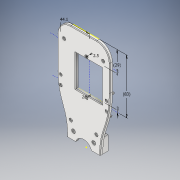
# Autodesk Inventor part: Sideplate
Saved by Autodesk Inventor 2019 (Build 230136000, 136)
## iProperties
Created: 2018-12-23
Part Number: Sideplate
Material: Generic
Document SubType Name: Modeling
Designer: Martin
Density: 1 g/cm^3
Appearance: Default
Mass: 44.7821 g
Surface Area: 242.538 cm^2
Volume: 44.7821 cm^3
Author: Martin
Autodesk Inventor part; units mm, degrees
ref_plane "YZ Plane" through (0, 0, 0) normal (1, 0, 0) x (0, 1, 0)
ref_plane "XZ Plane" through (0, 0, 0) normal (0, 1, 0) x (-1, 0, 0)
ref_plane "XY Plane" through (0, 0, 0) normal (0, 0, 1) x (1, 0, 0)
sketch "Sketch1" plane through (0, 0, 0) normal (0, 0, 1) x (1, 0, 0)
  line L0 (-21.25, 21.25) -> (21.25, 21.25)
  line L1 (21.25, 21.25) -> (21.25, -21.25)
  line L2 (21.25, -21.25) -> (-21.25, -21.25)
  line L3 (-21.25, -21.25) -> (-21.25, 21.25)
  line L4 (-21.25, 21.25) -> (21.25, -21.25) construction
  line L5 (21.25, 21.25) -> (-21.25, -21.25) construction
  circle A0 centre (0, 0) radius 11 construction
  circle A1 centre (0, 0) radius 12.5
  line L6 (-25.25, 3.5236) -> (25.25, 3.5236)
  line L7 (25.25, 3.5236) -> (25.25, 25.25)
  line L8 (25.25, 25.25) -> (-25.25, 25.25)
  line L9 (-25.25, 25.25) -> (-25.25, 3.5236)
  circle A2 centre (-15.5, 15.5) radius 1.5
  circle A3 centre (15.5, 15.5) radius 1.5
  point P0 (21.25, 3.5236)
  point P1 (-21.25, 3.5236)
  dimension "d0" = 42.5
  dimension "d1" = 42.5
  dimension "d2" = 22
  dimension "d3" = 25
  dimension "d4" = 4
  dimension "d5" = 4
  dimension "d6" = 4
  dimension "d7" = 3
  dimension "d8" = 3
  dimension "d9" = 15.5
  dimension "d10" = 15.5
  dimension "d11" = 15.5
  dimension "d12" = 15.5
  constraints: 20 end point, 4 centre point, 4 parallel, 4 point on line, 2 coincident, 2 horizontal, 2 midpoint, 2 perpendicular
  measures "d0" distance of L1.end L2.end
  measures "d1" distance of L0.end L1.end
  measures "d2" diameter of A0
  measures "d3" diameter of A1
  measures "d4" distance between parallel lines of L0 L8
  measures "d5" distance between parallel lines of L9 L3
  measures "d6" distance between parallel lines of L7 L1
  measures "d7" diameter of A3
  measures "d8" diameter of A2
  measures "d9" horizontal distance of A3.centre point (0, 0)
  measures "d10" horizontal distance of A3.centre point (0, 0)
  measures "d11" horizontal distance of A2.centre A0.centre
  measures "d12" horizontal distance of point (0, 0) A2.centre
extrude "Extrusion1" add sketch "Sketch1" along normal blind 4 contours L3 L6 L9 L8 L7 L1 L0 | L0 L1 L6 A1 L3 | A1 L6 picked at (3.04, 5.1985)
extrude "Extrusion3" add sketch "Sketch1" against normal blind 8 contours L3 L6 L9 L8 L7 L1 L0
sketch "Sketch2" plane through (0, 0, 4) normal (0, 0, 1) x (1, 0, 0)
  circle A0 centre (0, 0) radius 40 construction
  line L0 (-25.25, 3.5236) -> (25.25, 3.5236) construction
  line L1 (-25.25, 3.5236) -> (25.25, 3.5236) projected
  line L2 (-25.25, 3.5236) -> (25.25, 3.5236)
  line L3 (39.8445, 92.8978) -> (39.8445, 152.8119)
  line L4 (39.8445, 152.8119) -> (-39.8445, 152.8119)
  line L5 (-39.8445, 152.8119) -> (-39.8445, 82.8978)
  circle A1 centre (-15.5, 15.5) radius 1.5 projected
  circle A2 centre (-15.5, 15.5) radius 1.5
  circle A3 centre (15.5, 15.5) radius 1.5 projected
  circle A4 centre (15.5, 15.5) radius 1.5
  line L6 (25.25, 43.5236) -> (25.25, 3.5236) projected
  line L7 (25.25, 43.5236) -> (25.25, -31.0232) construction
  line L8 (-25.25, 25.25) -> (-25.25, -31.0232) construction
  line L9 (25.25, 3.5236) -> (25.25, 43.5236) projected
  line L10 (25.25, 3.5236) -> (25.25, 43.5236) construction
  line L11 (25.25, 43.5236) -> (39.8445, 43.5236) construction
  line L12 (39.8445, 43.5236) -> (39.8445, 92.8978) construction
  spline S0 degree 3 poles (25.25, 3.5236) (25.25, 43.5236) (39.8445, 43.5236) (39.8445, 92.8978) knots 1 1 1 1 2 2 2 2
  line L13 (-25.25, 3.5236) -> (-25.25, 43.5236) construction
  line L14 (-25.25, 43.5236) -> (-39.8445, 43.5236) construction
  line L15 (-39.8445, 43.5236) -> (-39.8445, 82.8978) construction
  spline S1 degree 3 poles (-25.25, 3.5236) (-25.25, 43.5236) (-39.8445, 43.5236) (-39.8445, 82.8978) knots 1 1 1 1 2 2 2 2
  line L16 (34.8445, 168.0706) -> (34.8445, -11.808) construction
  line L17 (-34.8445, 167.0543) -> (-34.8445, -11.808) construction
  line L18 (51.4064, 130.8119) -> (-51.1328, 130.8119) construction
  line L19 (29.8445, 167.0543) -> (29.8445, 90.5025) construction
  line L20 (-29.8445, 165.7121) -> (-29.8445, 89.1603) construction
  circle A5 centre (29.8445, 130.8119) radius 1.25
  circle A6 centre (-29.8445, 130.8119) radius 1.25
  point P0 (-11.9931, 3.5236)
  point P1 (-39.8445, 3.5236)
  point P2 (39.8445, 3.5236)
  dimension "d19" = 80
  dimension "d20" = 150
  dimension "d21" = 39.8445
  dimension "d33" = 40
  dimension "d34" = 40
  dimension "d35" = 40
  dimension "d36" = 39.8445
  dimension "d37" = 5
  dimension "d38" = 5
  dimension "d68" = 22
  dimension "d69" = 10
  dimension "d70" = 10
  dimension "d71" = 2.5
  dimension "d72" = 2.5
  constraints: 24 end point, 7 point on line, 5 centre point, 4 coincident, 4 collinear, 4 vertical, 3 parallel, 2 horizontal, 2 perpendicular, 2 point on circle, 8 other
  measures "d19" diameter of A0
  measures "d20" distance of L0.end L3.end
  measures "d21" distance from line of L3 A0.centre
  measures "d33" distance from line of L0 L14.end
  measures "d34" distance from line of L0 L11.end
  measures "d35" distance from line of L0 L6.start
  measures "d36" distance from line of L5 point (0, 0)
  measures "d37" distance between parallel lines of L3 L16
  measures "d38" distance between parallel lines of L5 L17
  measures "d68" distance between parallel lines of L18 L4
  measures "d69" distance between parallel lines of L19 L3
  measures "d70" distance between parallel lines of L5 L20
  measures "d71" diameter of A5
  measures "d72" diameter of A6
extrude "Extrusion4" add sketch "Sketch2" against normal blind 4 contours S1 L5 L4 L3 S0 L1 | A5 | A6
fillet "Fillet1" radius 20 2 edges at (-39.8445, 152.8119, 2) (39.8445, 152.8119, 2)
sketch "Sketch3" plane through (0, 0, 0) normal (0, 0, -1) x (-1, 0, 0)
  line L0 (-40.0079, 28.25) -> (78.3012, 28.25) construction
  line L1 (25.25, 25.25) -> (-25.25, 25.25) projected
  line L2 (-19.5, 51.7245) -> (-19.5, -25.7194) construction
  line L3 (19.5, 50.7243) -> (19.5, -26.4338) construction
  circle A0 centre (-19.5, 28.25) radius 1.25
  circle A1 centre (19.5, 28.25) radius 1.25
  point P0 (0, 0)
  dimension "d26" = 3
  dimension "d27" = 19.5
  dimension "d28" = 19.5
  dimension "d29" = 2.5
  dimension "d30" = 2.5
  constraints: 6 end point, 4 point on line, 2 centre point, 2 vertical, 1 horizontal
  measures "d26" distance between parallel lines of L0 L1
  measures "d27" distance from line of point (0, 0) L2
  measures "d28" distance from line of L3 point (0, 0)
  measures "d29" diameter of A0
  measures "d30" diameter of A1
extrude "Extrusion5" cut sketch "Sketch3" against normal blind 10
sketch "Sketch4" plane through (0, 0, 0) normal (0, 0, -1) x (-1, 0, 0)
  line L0 (-34.8445, 174.3908) -> (-34.8445, -4.6748) construction
  line L1 (34.8445, 172.891) -> (34.8445, -6.1746) construction
  line L2 (39.8445, 174.885) -> (39.8445, -4.1806) construction
  line L3 (39.8445, 82.8978) -> (39.8445, 132.8119) projected
  line L4 (-39.8445, 132.8119) -> (-39.8445, 92.8978) projected
  line L5 (-58.077, 152.8119) -> (62.4518, 152.8119) construction
  line L6 (19.8445, 152.8119) -> (-19.8445, 152.8119) projected
  line L7 (-60.7578, 80.8119) -> (59.771, 80.8119) construction
  line L8 (-61.2028, 66.8119) -> (59.326, 66.8119) construction
  circle A0 centre (-34.8445, 80.8119) radius 1
  circle A1 centre (-34.8445, 66.8119) radius 1
  circle A2 centre (34.8445, 80.8119) radius 1
  circle A3 centre (34.8445, 66.8119) radius 1
  line L9 (-29.8445, 176.1827) -> (-29.8445, -2.8829) construction
  line L10 (29.8445, 178.0117) -> (29.8445, -1.0539) construction
  line L11 (-58.5074, 88.8119) -> (62.0214, 88.8119) construction
  line L12 (-58.4589, 58.8119) -> (62.0699, 58.8119) construction
  line L13 (-39.8445, 88.8119) -> (-29.8445, 88.8119) construction
  line L14 (-29.8445, 88.8119) -> (-29.8445, 58.8119) construction
  line L15 (-29.8445, 58.8119) -> (-36.5289, 58.8119) construction
  line L16 (-36.5289, 58.7119) -> (-29.7445, 58.7119)
  line L17 (-29.7445, 58.7119) -> (-29.7445, 88.9119)
  line L18 (-29.7445, 88.9119) -> (-39.7987, 88.9119)
  line L19 (-39.8276, 90.9119) -> (-27.7445, 90.9119)
  line L20 (-27.7445, 56.7119) -> (-36.0331, 56.7119)
  line L21 (-36.5289, 58.7119) -> (-36.0331, 56.7119)
  line L22 (-39.8445, 176.1815) -> (-39.8445, 90.9119) construction
  line L23 (-39.8445, 88.9119) -> (-39.8445, -2.8841) construction
  line L24 (-39.8276, 90.9119) -> (-39.7987, 88.9119)
  line L25 (0, 0) -> (0, 162.0516)
  circle A4 centre (34.8445, 80.8119) radius 1
  circle A5 centre (34.8445, 66.8119) radius 1
  line L26 (39.8445, 88.8119) -> (29.8445, 88.8119) construction
  line L27 (29.8445, 88.8119) -> (29.8445, 58.8119) construction
  line L28 (29.8445, 58.8119) -> (36.5289, 58.8119) construction
  line L29 (36.5289, 58.7119) -> (29.7445, 58.7119)
  line L30 (29.7445, 58.7119) -> (29.7445, 88.9119)
  line L31 (29.7445, 88.9119) -> (39.7987, 88.9119)
  line L32 (39.8276, 90.9119) -> (27.7445, 90.9119)
  line L33 (27.7445, 90.9119) -> (27.7445, 56.7119)
  line L34 (27.7445, 56.7119) -> (36.0331, 56.7119)
  line L35 (36.5289, 58.7119) -> (36.0331, 56.7119)
  line L36 (39.8276, 90.9119) -> (39.7987, 88.9119)
  line L37 (0, 66.8119) -> (5.554, 66.8119)
  line L38 (12.2555, 72.8119) -> (12.2555, 120.8119)
  line L39 (12.2555, 120.8119) -> (-27.7445, 120.8119)
  line L40 (-27.7445, 120.8119) -> (-27.7445, 66.8119)
  line L41 (-27.7445, 72.8119) -> (12.2555, 72.8119)
  line L42 (-27.7445, 90.9119) -> (-27.7445, 72.8119)
  line L43 (-27.7445, 66.8119) -> (-27.7445, 56.7119)
  point P0 (-29.8445, 82.3994)
  point P1 (-29.8445, 68.3994)
  point P2 (29.8445, 83.9869)
  point P3 (29.8445, 69.9869)
  point P4 (-33.257, 88.8119)
  point P5 (36.432, 88.8119)
  point P6 (-33.257, 58.8119)
  point P7 (36.432, 58.8119)
  point P8 (39.8445, 92.8978)
  point P9 (29.8445, 82.3994)
  point P10 (29.8445, 68.3994)
  point P11 (33.257, 88.8119)
  point P12 (33.257, 58.8119)
  point P13 (39.8445, 88.9119)
  point P14 (39.8445, 90.9119)
  dimension "d40" = 5
  dimension "d41" = 72
  dimension "d42" = 14
  dimension "d43" = 2
  dimension "d44" = 2
  dimension "d45" = 2
  dimension "d46" = 2
  dimension "d49" = 5
  dimension "d50" = 5
  dimension "d51" = 8
  dimension "d52" = 8
  dimension "d53" = 0.1
  dimension "d61" = 32
  dimension "d62" = 80
  dimension "d63" = 40
  constraints: 82 end point, 26 point on line, 19 symmetric about line, 8 vertical, 6 centre point, 6 horizontal, 4 collinear, 2 parallel, 2 perpendicular, 3 other
  measures "d40" distance between parallel lines of L2 L1
  measures "d41" distance between parallel lines of L7 L5
  measures "d42" distance between parallel lines of L8 L7
  measures "d43" diameter of A0
  measures "d44" diameter of A1
  measures "d45" diameter of A2
  measures "d46" diameter of A3
  measures "d49" distance between parallel lines of L9 L0
  measures "d50" distance between parallel lines of L1 L10
  measures "d51" distance between parallel lines of L7 L11
  measures "d52" distance from line of L12 L8.end
  measures "d53" distance between parallel lines of L14 L17
  measures "d61" distance between parallel lines of L39 L5
  measures "d62" distance between parallel lines of L41 L5
  measures "d63" distance of L38.end L39.end
extrude "Extrusion6" cut sketch "Sketch4" against normal blind 10 contours A0 | A1 | A2 | A3
extrude "Extrusion7" add sketch "Sketch4" along normal blind 3 contours L16 L17 L18 L24 L19 L40 L43 L20 L21
extrude "Extrusion8" add sketch "Sketch4" along normal blind 3 contours L35 L34 L33 L32 L36 L31 L30 L29
extrude "Extrusion9" cut sketch "Sketch4" against normal blind 10 contours L40 L39 L25 L41 | L25 L39 L38 L41
fillet "Fillet3" radius 1 4 edges at (-12.2555, 96.8119, 4) (7.7445, 120.8119, 4) (27.7445, 96.8119, 4) (7.7445, 72.8119, 4)
fillet "Fillet4" radius 1 7 edges at (-33.9866, 146.954, 4) (0, 152.8119, 4) (33.9866, 146.954, 4) (39.8445, 112.8548, 4) (32.5473, 44.6953, 4) (-32.5473, 43.4453, 4) (-39.8445, 107.8548, 4)
extrude "Extrusion10" cut sketch "Sketch1" along normal blind 10 contours L6 A1 | A1 L6
extrude "Extrusion11" cut sketch "Sketch2" against normal blind 10 contours A5 | A6
sketch "Sketch5" plane through (0, 0, 0) normal (0, 0, -1) x (-1, 0, 0)
  line L0 (-4.2555, 145.2957) -> (-4.2555, 45.6787) construction
  line L1 (39.8445, 82.8978) -> (39.8445, 132.8119) projected
  line L2 (-46.5936, 123.8119) -> (55.7766, 123.8119) construction
  line L3 (-27.7445, 120.8119) -> (12.2555, 120.8119) construction
  line L4 (-50.3875, 69.8119) -> (51.9828, 69.8119) construction
  line L5 (12.2555, 72.8119) -> (-27.7445, 72.8119) construction
  circle A0 centre (-4.2555, 123.8119) radius 1.25
  circle A1 centre (-4.2555, 69.8119) radius 1.25
  line L6 (19.8445, 152.8119) -> (-19.8445, 152.8119) projected
  point P0 (0, 0)
  dimension "d75" = 44.1
  dimension "d77" = 3
  dimension "d78" = 3
  dimension "d79" = 2.5
  dimension "d80" = 2.5
  dimension "d83" = 29
  dimension "d84" = 83
  constraints: 6 end point, 4 point on line, 2 centre point, 2 horizontal, 1 vertical
  measures "d75" distance between parallel lines of L1 L0
  measures "d77" distance between parallel lines of L2 L3
  measures "d78" distance between parallel lines of L4 L5
  measures "d79" diameter of A0
  measures "d80" diameter of A1
  measures "d83" distance between parallel lines of L2 L6
  measures "d84" distance between parallel lines of L4 L6
extrude "Extrusion12" cut sketch "Sketch5" against normal blind 10
sketch "Sketch6" plane through (0, 0, 4) normal (0, 0, 1) x (1, 0, 0)
  circle A0 centre (29.8445, 130.8119) radius 1.25 projected
  circle A1 centre (29.8445, 130.8119) radius 2.5
  circle A2 centre (-29.8445, 130.8119) radius 1.25 projected
  circle A3 centre (-29.8445, 130.8119) radius 2.5
  circle A4 centre (4.2555, 123.8119) radius 1.25 projected
  circle A5 centre (4.2555, 123.8119) radius 2.5
  circle A6 centre (4.2555, 69.8119) radius 1.25 projected
  circle A7 centre (4.2555, 69.8119) radius 2.5
  circle A8 centre (-19.5, 28.25) radius 1.25 projected
  circle A9 centre (-19.5, 28.25) radius 2.5
  circle A10 centre (19.5, 28.25) radius 1.25 projected
  circle A11 centre (19.5, 28.25) radius 2.5
  circle A12 centre (15.5, 15.5) radius 1.5 projected
  circle A13 centre (15.5, 15.5) radius 3
  circle A14 centre (-15.5, 15.5) radius 1.5 projected
  circle A15 centre (-15.5, 15.5) radius 3
  circle A16 centre (34.8445, 80.8119) radius 1 projected
  circle A17 centre (34.8445, 80.8119) radius 2.25
  circle A18 centre (34.8445, 66.8119) radius 1 projected
  circle A19 centre (34.8445, 66.8119) radius 2.25
  circle A20 centre (-34.8445, 80.8119) radius 1 projected
  circle A21 centre (-34.8445, 80.8119) radius 2.25
  circle A22 centre (-34.8445, 66.8119) radius 1 projected
  circle A23 centre (-34.8445, 66.8119) radius 2.25
  point P0 (0, 0)
  dimension "d85" = 5
  dimension "d86" = 5
  dimension "d87" = 5
  dimension "d88" = 5
  dimension "d89" = 5
  dimension "d90" = 5
  dimension "d91" = 6
  dimension "d92" = 6
  dimension "d93" = 4.5
  dimension "d94" = 4.5
  dimension "d95" = 4.5
  dimension "d96" = 4.5
  constraints: 12 centre point, 12 coincident
  measures "d85" diameter of A1
  measures "d86" diameter of A3
  measures "d87" diameter of A5
  measures "d88" diameter of A7
  measures "d89" diameter of A9
  measures "d90" diameter of A11
  measures "d91" diameter of A13
  measures "d92" diameter of A15
  measures "d93" diameter of A17
  measures "d94" diameter of A19
  measures "d95" diameter of A21
  measures "d96" diameter of A23
extrude "Extrusion13" cut sketch "Sketch6" against normal blind 1
equation "\"d1\" = d0"
equation "\"d5\" = d4"
equation "\"d6\" = d4"
equation "\"d8\" = d7"
equation "\"d11\" = d9"
equation "\"d12\" = d10"
equation "\"d21\" = d36"
equation "\"d34\" = d33"
equation "\"d35\" = d33"
equation "\"d38\" = d37"
equation "\"d28\" = d27"
body "Solid1"
